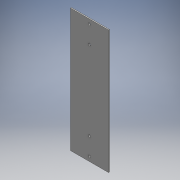
# Autodesk Inventor part: Part3
Saved by Autodesk Inventor 2016 (Build 200138000, 138)
## iProperties
Created: 2016-11-05
Part Number: Part3
Material: 一般
Document SubType Name: Modeling
Designer: 宏太
Density: 1 g/cm^3
Appearance: 既定
Mass: 41.4429 g
Surface Area: 429.286 cm^2
Volume: 41.4429 cm^3
Author: 宏太
Autodesk Inventor part; units mm, degrees
ref_plane "YZ Plane" through (0, 0, 0) normal (1, 0, 0) x (0, 1, 0)
ref_plane "XZ Plane" through (0, 0, 0) normal (0, 1, 0) x (-1, 0, 0)
ref_plane "XY Plane" through (0, 0, 0) normal (0, 0, 1) x (1, 0, 0)
sketch "スケッチ1" plane through (0, 0, 0) normal (0, 1, 0) x (-1, 0, 0)
  line L0 (0, 0) -> (80, 0)
  line L1 (80, 0) -> (80, -260)
  line L2 (80, -260) -> (0, -260)
  line L3 (0, -260) -> (0, 0)
  dimension "d0" = 80
  dimension "d1" = 260
  constraints: 8 end point, 2 parallel, 1 horizontal, 1 perpendicular
  measures "d0" distance of L1.end L2.end
  measures "d1" distance of L0.end L1.end
extrude "押し出し1" add sketch "スケッチ1" along normal blind 2
sketch "スケッチ2" plane through (0, 0, 0) normal (0, -1, 0) x (1, 0, 0)
  circle A0 centre (-40, -9.5) radius 2.5
  line L0 (0, -260) -> (0, 0) projected
  line L1 (0, 0) -> (-80, 0) projected
  circle A1 centre (-40, -46.5) radius 2.5
  circle A2 centre (-40, -250.5) radius 2.5
  circle A3 centre (-40, -213.5) radius 2.5
  line L2 (-80, -260) -> (0, -260) projected
  dimension "d4" = 5
  dimension "d6" = 40
  dimension "d7" = 9.5
  dimension "d8" = 5
  dimension "d10" = 40
  dimension "d11" = 5
  dimension "d12" = 5
  dimension "d13" = 40
  dimension "d14" = 9.5
  dimension "d15" = 40
  dimension "d28" = 37
  dimension "d29" = 37
  constraints: 4 centre point
  measures "d4" diameter of A0
  measures "d6" distance from line of L0 A0.centre
  measures "d7" distance from line of L1 A0.centre
  measures "d8" diameter of A1
  measures "d10" distance from line of L0 A1.centre
  measures "d11" diameter of A2
  measures "d12" diameter of A3
  measures "d13" distance from line of L0 A2.centre
  measures "d14" distance from line of L2 A2.centre
  measures "d15" distance from line of L0 A3.centre
  measures "d28" distance of A1.centre A0.centre
  measures "d29" distance of A3.centre A2.centre
extrude "押し出し2" cut sketch "スケッチ2" against normal blind 10
